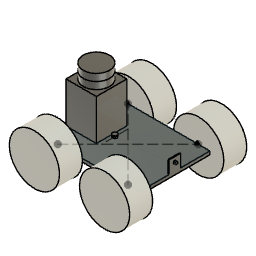
smt_model_gazebo (Autodesk Fusion 360 design; units mm, degrees)
Autodesk Fusion 360 part; units mm, degrees
note: some values were not read from the file. Set by a fixed rule: which sketch regions a step uses.
sketch "Sketch1" plane through (0, 0, 0) normal (0, 0, 1) x (1, 0, 0) in component "base_link"
  line L0 (-100, -75) -> (100, -75)
  line L1 (100, -75) -> (100, 75)
  line L2 (100, 75) -> (-100, 75)
  line L3 (-100, 75) -> (-100, -75)
  line L4 (-100, -75) -> (100, 75) construction
  line L5 (100, -75) -> (-100, 75) construction
  dimension "d13" = 200
  dimension "d14" = 150
  constraint horizontal L0
  constraint perpendicular L0 L1
  constraint parallel L0 L2
  constraint parallel L1 L3
  constraint coincident L4 origin
  constraint coincident L5 origin
  measures "d13" distance of L1.end L2.end
  measures "d14" distance of L0.end L1.end
extrude "Extrude1" add sketch "Sketch1" along normal blind 7 from surface at 50 makes body 1 in component "base_link"
sketch "Sketch5" plane through (0, 75, 0) normal (0, 1, 0) x (-1, 0, 0) in component "base_link"
  line L0 (-100, 50) -> (100, 50)
  line L1 (100, 50) -> (100, 57)
  line L2 (100, 57) -> (-100, 57)
  line L3 (-100, 57) -> (-100, 50)
  line L4 (-100, 53.5) -> (100, 53.5) construction
  line L5 (75, 57) -> (75, 50) construction
  line L6 (0, 57) -> (0, 0) construction
  line L7 (-75, 57) -> (-75, 50) construction
  circle A0 centre (75, 53.5) radius 3.5
  circle A1 centre (-75, 53.5) radius 3.5
  dimension "d34" = 150
  constraint midpoint L3 L4.start
  constraint midpoint L1 L4.end
  constraint coincident L2 L5.start
  constraint coincident L0 L5.end
  constraint perpendicular L0 L5
  constraint midpoint L2 L6.start
  constraint coincident L6.end origin
  constraint coincident L2 L7.start
  constraint coincident L0 L7.end
  constraint perpendicular L0 L7
  constraint symmetric L5 L6 L7
  constraint midpoint L5 A0.centre
  constraint coincident L5.end A0
  constraint midpoint L7 A1.centre
  constraint coincident L7.end A1
  measures "d34" distance of L5 L7
extrude "Extrude4" add sketch "Sketch5" along normal blind 1 contours A1 | A0 bodies 1 in component "base_link"
mirror "Mirror1" about plane through (0, 0, 0) normal (0, 1, 0) of "Extrude4" in component "base_link"
sketch "Sketch2" plane through (0, 0, 57) normal (0, 0, 1) x (-1, 0, 0) in component "base_link"
  line L0 (100, -75) -> (100, 75)
  line L1 (100, 75) -> (75, 75)
  line L2 (-100, 75) -> (-100, -75)
  line L3 (-100, -75) -> (-75, -75)
  line L4 (67.5, -75) -> (67.5, 75) construction
  line L5 (100, 32.5) -> (35, 32.5)
  line L6 (35, 32.5) -> (35, -32.5)
  line L7 (35, -32.5) -> (100, -32.5)
  line L8 (100, -32.5) -> (100, 32.5)
  line L9 (100, 32.5) -> (35, -32.5) construction
  line L10 (35, 32.5) -> (100, -32.5) construction
  circle A0 centre (67.5, 0) radius 28
  line L11 (75, 75) -> (-75, 75)
  line L12 (-75, 75) -> (-100, 75)
  line L13 (-75, -75) -> (75, -75)
  line L14 (75, -75) -> (100, -75)
  point P0 (67.5, 0)
  dimension "d24" = 32.5
  dimension "d25" = 65
  dimension "d26" = 56
  constraint coincident L3 L4.start
  constraint coincident L1 L4.end
  constraint perpendicular L1 L4
  constraint horizontal L5
  constraint perpendicular L5 L6
  constraint parallel L5 L7
  constraint parallel L6 L8
  constraint coincident L9 P0
  constraint coincident L10 P0
  constraint coincident L0 L5.start
  constraint midpoint L4 P0
  constraint coincident P0 A0.centre
  measures "d24" distance of L0 L4
  measures "d25" distance of L5.end L6.end
  measures "d26" diameter of A0
extrude "Extrude2" add sketch "Sketch2" along normal blind 87 contours L0 L5 L6 L7 L8 | A0 bodies 1 in component "base_link"
extrude "Extrude3" add sketch "Sketch2" along normal blind 15 from surface at 87 contours A0 bodies 1 in component "base_link"
extrude "Extrude1'" add 1 faces at (-73.8289, 14.0977, 159) along direction (0, 0, 1) blind 15 separate body on bodies 1 makes body 2 in component "lidar"
sketch "Sketch1 (2)" plane through (0, -76, 0) normal (0, -1, 0) x (1, 0, 0) in component "wheel_right_back"
  circle A0 centre (-75, 53.5) radius 3.5
  circle A1 centre (-75, 53.5) radius 53.5
  dimension "d44" = 107
  constraint concentric A0 A1
  measures "d44" diameter of A1
extrude "Extrude1''" add sketch "Sketch1 (2)" along normal blind 49 separate body contours A0 | A1 makes body 3 in component "wheel_right_back"
sketch "Sketch1 (3)" plane through (0, -76, 0) normal (0, -1, 0) x (1, 0, 0) in component "wheel_right_front"
  circle A0 centre (75, 53.5) radius 3.5
  circle A1 centre (75, 53.5) radius 53.5
  dimension "d47" = 107
  constraint concentric A0 A1
  measures "d47" diameter of A1
extrude "Extrude1'''" add sketch "Sketch1 (3)" along normal blind 49 separate body contours A0 | A1 makes body 4 in component "wheel_right_front"
mirror "MirrorComponent2" about plane through (0, 0, 0) normal (0, 0, 1) of bodies 3 makes body 5 in component "wheel_left_back"
mirror "MirrorComponent2'" about plane through (0, 0, 0) normal (0, 0, 1) of bodies 4 makes body 6 in component "wheel_left_front"
sketch "Sketch6" plane through (0, 0, 57) normal (0, 0, 1) x (-1, 0, 0) in component "base_link"
  line L0 (35, 32.5) -> (100, 32.5)
  line L1 (100, 32.5) -> (100, 75)
  line L2 (100, 75) -> (75, 75)
  line L3 (75, 75) -> (-75, 75)
  line L4 (-75, 75) -> (-100, 75)
  line L5 (-100, 75) -> (-100, -75)
  line L6 (-100, -75) -> (-75, -75)
  line L7 (-75, -75) -> (75, -75)
  line L8 (75, -75) -> (100, -75)
  line L9 (100, -75) -> (100, -32.5)
  line L10 (100, -32.5) -> (35, -32.5)
  line L11 (35, -32.5) -> (35, 32.5)
  line L12 (-100, 12.5) -> (-98, 12.5)
  line L13 (-98, 12.5) -> (-98, -12.5)
  line L14 (-98, -12.5) -> (-100, -12.5)
  line L15 (-100, -12.5) -> (-100, 12.5)
  line L16 (35, 0) -> (100, 0) construction
  dimension "d70" = 2
  dimension "d71" = 25
  constraint horizontal L12
  constraint vertical L13
  constraint horizontal L14
  constraint vertical L15
  constraint coincident L5 L12.start
  constraint midpoint L11 L16.start
  constraint perpendicular L11 L16
  constraint symmetric L12 L14 L16
  measures "d70" distance of L12.start L12.end
  measures "d71" distance of L12.end L13.end
extrude "Extrude5" add sketch "Sketch6" along normal blind 27 contours L5 L12 L13 L14 L15 bodies 1 in component "base_link"
sketch "Sketch1 (4)" plane through (100, 0, 0) normal (1, 0, 0) x (0, 1, 0) in component "cam"
  line L0 (-75, 50) -> (75, 50)
  line L1 (75, 50) -> (75, 57)
  line L2 (75, 57) -> (12.5, 57)
  line L3 (12.5, 57) -> (12.5, 84)
  line L4 (12.5, 84) -> (-12.5, 84)
  line L5 (-12.5, 84) -> (-12.5, 57)
  line L6 (-12.5, 57) -> (-75, 57)
  line L7 (-75, 57) -> (-75, 50)
  circle A0 centre (0, 74) radius 3
  dimension "d74" = 6
  dimension "d75" = 12.5
  dimension "d76" = 17
  measures "d74" diameter of A0
  measures "d75" distance of L3 A0.centre
  measures "d76" distance of L6 A0.centre
extrude "Extrude2'" add sketch "Sketch1 (4)" along normal blind 3 from surface at 0.5 separate body contours A0 makes body 7 in component "cam"
sketch "Sketch7" plane through (100, 0, 0) normal (1, 0, 0) x (0, 1, 0) in component "base_link"
  circle A0 centre (0, 74) radius 3
  circle A1 centre (0, 74) radius 3
  dimension "d83" = 6
  constraint concentric A0 A1
  measures "d83" diameter of A1
extrude "Extrude6" add sketch "Sketch1 (4)" along normal blind 0.5 contours A0 bodies 1 in component "base_link"
sketch "Sketch3" plane through (0, 0, 57) normal (0, 0, 1) x (-1, 0, 0)
  line L0 (-100, 12.5) -> (-98, 12.5)
  line L1 (-98, 12.5) -> (-98, -12.5)
  line L2 (-98, -12.5) -> (-100, -12.5)
  line L3 (-100, -12.5) -> (-100, -75)
  line L4 (-100, -75) -> (-75, -75)
  line L5 (-75, -75) -> (75, -75)
  line L6 (75, -75) -> (100, -75)
  line L7 (100, -75) -> (100, -32.5)
  line L8 (100, -32.5) -> (35, -32.5)
  line L9 (35, -32.5) -> (35, 32.5)
  line L10 (35, 32.5) -> (100, 32.5)
  line L11 (100, 32.5) -> (100, 75)
  line L12 (100, 75) -> (75, 75)
  line L13 (75, 75) -> (-75, 75)
  line L14 (-75, 75) -> (-100, 75)
  line L15 (-100, 75) -> (-100, 12.5)
  line L16 (-75, 75) -> (75, -75) construction
  line L17 (75, 75) -> (-75, -75) construction
  line L18 (28, -28) -> (28, 28) construction
  dimension "d99" = 28
  constraint coincident L13.end L14.start
  constraint coincident L5.end L6.start
  constraint coincident L12.end L13.start
  constraint coincident L4.end L5.start
  constraint coincident L16 L18.start
  constraint coincident L17 L18.end
  constraint perpendicular L8 L18
  measures "d99" distance of origin L18
sketch "Sketch8" plane through (0, 0, 57) normal (0, 0, 1) x (-1, 0, 0) in component "base_link"
  line L0 (-100, 12.5) -> (-98, 12.5)
  line L1 (-98, 12.5) -> (-98, -12.5)
  line L2 (-98, -12.5) -> (-100, -12.5)
  line L3 (-100, -12.5) -> (-100, -75)
  line L4 (-100, -75) -> (-75, -75)
  line L5 (-75, -75) -> (75, -75)
  line L6 (75, -75) -> (100, -75)
  line L7 (100, -75) -> (100, -32.5)
  line L8 (100, -32.5) -> (35, -32.5)
  line L9 (35, -32.5) -> (35, 32.5)
  line L10 (35, 32.5) -> (100, 32.5)
  line L11 (100, 32.5) -> (100, 75)
  line L12 (100, 75) -> (75, 75)
  line L13 (75, 75) -> (-75, 75)
  line L14 (-75, 75) -> (-100, 75)
  line L15 (-100, 75) -> (-100, 12.5)
  line L16 (35, 0) -> (-98, 0) construction
  line L17 (0, -75) -> (0, 75) construction
  line L18 (-75, 75) -> (75, -75) construction
  line L19 (75, 75) -> (-75, -75) construction
  line L20 (28, -28) -> (28, 28)
  circle A0 centre (28, 0) radius 5
  dimension "d102" = 10
  constraint midpoint L9 L16.start
  constraint midpoint L1 L16.end
  constraint midpoint L5 L17.start
  constraint midpoint L13 L17.end
  constraint midpoint L20 A0.centre
  measures "d102" diameter of A0
extrude "Extrude8" add sketch "Sketch8" along normal blind 3 contours L20 A0 | L20 A0 bodies 1 in component "base_link"
extrude "Extrude2''" add 1 faces at (-30.0726, -1.6249, 60) along direction (0, 0, 1) blind 2 separate body on bodies 1 makes body 8 in component "IMU"
component "base_link" placed x (1, 0, 0) y (0, 1, 0) z (0, 0, 1) at (0, 0, 0)
component "lidar" placed x (1, 0, 0) y (0, 1, 0) z (0, 0, 1) at (0, 0, 0)
component "wheel_right_back" placed x (1, 0, 0) y (0, 1, 0) z (0, 0, 1) at (0, 0, 0)
component "wheel_right_front" placed x (1, 0, 0) y (0, 1, 0) z (0, 0, 1) at (0, 0, 0)
component "wheel_left_back" placed x (1, 0, 0) y (0, -1, 0) z (0, 0, -1) at (0, 0, 0)
component "wheel_left_front" placed x (1, 0, 0) y (0, -1, 0) z (0, 0, -1) at (0, 0, 0)
component "cam" placed x (1, 0, 0) y (0, 1, 0) z (0, 0, 1) at (0, 0, 0)
component "IMU" placed x (1, 0, 0) y (0, 1, 0) z (0, 0, 1) at (0, 0, 0)
